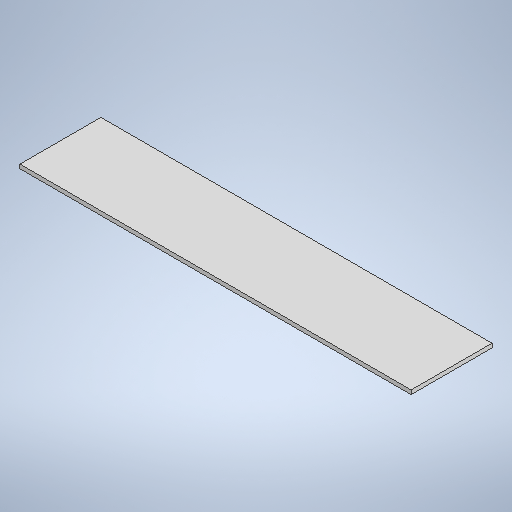
# Autodesk Inventor part: XaxisScaleMount
Saved by Autodesk Inventor 2025 (Build 290162010, 162A)
## iProperties
Created: 2024-08-21
Part Number: XaxisScaleMount
Material: Generic
Document SubType Name: Modeling
Designer: max_d
Density: 1 g/cm^3
Appearance: Default
Author: max_d
Autodesk Inventor part; units mm, degrees
ref_plane "YZ Plane" through (0, 0, 0) normal (1, 0, 0) x (0, 1, 0)
ref_plane "XZ Plane" through (0, 0, 0) normal (0, 1, 0) x (-1, 0, 0)
ref_plane "XY Plane" through (0, 0, 0) normal (0, 0, 1) x (1, 0, 0)
sketch "Sketch1" plane through (0, 0, 0) normal (1, 0, 0) x (0, 1, 0)
  line L0 (-1.5, 30) -> (1.5, 30)
  line L1 (1.5, 30) -> (1.5, -30)
  line L2 (1.5, -30) -> (-1.5, -30)
  line L3 (-1.5, -30) -> (-1.5, 30)
  line L4 (-1.5, 30) -> (1.5, -30) construction
  line L5 (1.5, 30) -> (-1.5, -30) construction
  point P0 (0, 0)
  dimension "d0" = 3
  dimension "d1" = 60
  constraints: 12 end point, 2 midpoint, 2 parallel, 1 horizontal, 1 perpendicular
  measures "d0" distance of L1.end L2.end
  measures "d1" distance of L0.end L1.end
extrude "Extrusion1" add sketch "Sketch1" along normal mid plane 290
body "Solid1"
